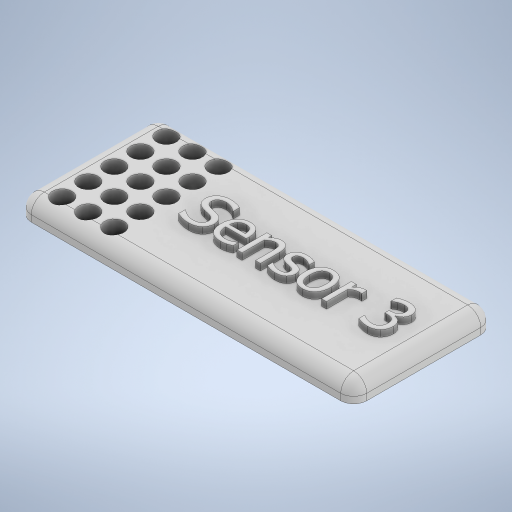
# Autodesk Inventor part: sensor3
Saved by Autodesk Inventor 2024 (Build 280153000, 153)
## iProperties
Created: 2024-03-06
Part Number: sensor3
Material: Generic
Document SubType Name: Modeling
Designer: quinten
Density: 1 g/cm^3
Appearance: Default
Author: quinten
Autodesk Inventor part; units mm, degrees
ref_plane "YZ Plane" through (0, 0, 0) normal (1, 0, 0) x (0, 1, 0)
ref_plane "XZ Plane" through (0, 0, 0) normal (0, 1, 0) x (-1, 0, 0)
ref_plane "XY Plane" through (0, 0, 0) normal (0, 0, 1) x (1, 0, 0)
sketch "Sketch1" plane through (0, 0, 0) normal (0, 1, 0) x (-1, 0, 0)
  line L0 (0, 0) -> (51.5, 0)
  line L1 (51.5, 0) -> (51.5, -21.5)
  line L2 (51.5, -21.5) -> (0, -21.5)
  line L3 (0, -21.5) -> (0, 0)
  line L4 (51.5, -10.75) -> (0, -10.75) construction
  line L5 (47.5, 0) -> (47.5, -21.5) construction
  circle A0 centre (47.5, -2.75) radius 1.5
  circle A1 centre (47.5, -10.75) radius 1.5
  circle A2 centre (47.5, -6.75) radius 1.5
  circle A3 centre (47.5, -14.75) radius 1.5
  circle A4 centre (47.5, -18.75) radius 1.5
  circle A5 centre (43.5, -2.75) radius 1.5
  circle A6 centre (43.5, -6.75) radius 1.5
  circle A7 centre (43.5, -10.75) radius 1.5
  circle A8 centre (43.5, -14.75) radius 1.5
  circle A9 centre (43.5, -18.75) radius 1.5
  circle A10 centre (39.5, -2.75) radius 1.5
  circle A11 centre (39.5, -6.75) radius 1.5
  circle A12 centre (39.5, -10.75) radius 1.5
  circle A13 centre (39.5, -14.75) radius 1.5
  circle A14 centre (39.5, -18.75) radius 1.5
  dimension "d0" = 51.5
  dimension "d1" = 21.5
  dimension "d2" = 4
  dimension "d3" = 3
  dimension "d4" = 3
  dimension "d5" = 3
  dimension "d6" = 3
  dimension "d7" = 3
  dimension "d8" = 4
  dimension "d9" = 4
  dimension "d10" = 4
  dimension "d11" = 4
  dimension "d14" = 4
  constraints: 15 centre point, 12 end point, 6 point on line, 3 midpoint, 2 horizontal, 2 parallel, 2 perpendicular, 20 other
  measures "d0" distance of L1.end L2.end
  measures "d1" distance of L0.end L1.end
  measures "d2" distance between parallel lines of L1 L5
  measures "d3" diameter of A0
  measures "d4" diameter of A1
  measures "d5" diameter of A2
  measures "d6" diameter of A3
  measures "d7" diameter of A4
  measures "d8" distance of A1.centre A3.centre
  measures "d9" distance of A3.centre A4.centre
  measures "d10" distance of A1.centre A2.centre
  measures "d11" distance of A2.centre A0.centre
  measures "d14" distance of A0.centre A5.centre
extrude "Extrusion1" add sketch "Sketch1" along normal blind 3
fillet "Fillet1" radius 2 8 edges at (0, 1.5, 0) (-25.75, 3, 0) (0, 3, -10.75) (0, 1.5, -21.5) (-25.75, 3, -21.5) (-51.5, 3, -10.75) (-51.5, 1.5, 0) (-51.5, 1.5, -21.5)
sketch "Sketch2" plane through (0, 3, 0) normal (0, 1, 0) x (1, 0, 0)
  line L0 (-35.6591, 14.3268) -> (-1.7873, 14.3268) construction
  line L1 (-1.7873, 14.3268) -> (-1.7873, 6.1649) construction
  line L2 (-1.7873, 6.1649) -> (-35.6591, 6.1649) construction
  line L3 (-35.6591, 6.1649) -> (-35.6591, 14.3268) construction
  spline S0 degree 2 poles (-33.3407, 7.9895) (-34.0031, 7.9895) (-34.9325, 8.2663) (-35.3428, 8.464) knots 0 0 0 1 2 2 2
  line L4 (-35.3428, 8.464) -> (-35.3428, 9.4823)
  line L5 (-35.3428, 9.4823) -> (-35.2834, 9.4823)
  spline S1 degree 2 poles (-35.2834, 9.4823) (-34.883, 9.1067) (-33.8697, 8.6914) (-33.4, 8.6914) knots 0 0 0 1 2 2 2
  spline S2 degree 2 poles (-33.4, 8.6914) (-32.7278, 8.6914) (-32.0406, 9.25) (-32.0406, 9.7097) knots 0 0 0 1 2 2 2
  spline S3 degree 2 poles (-32.0406, 9.7097) (-32.0406, 10.0755) (-32.4015, 10.5303) (-32.792, 10.644) knots 0 0 0 1 2 2 2
  spline S4 degree 2 poles (-32.792, 10.644) (-33.0738, 10.7231) (-33.5434, 10.8319) (-33.8944, 10.9208) knots 0 0 0 1 2 2 2
  spline S5 degree 2 poles (-33.8944, 10.9208) (-34.2107, 11.0049) (-34.71, 11.257) (-34.9028, 11.4597) knots 0 0 0 1 2 2 2
  spline S6 degree 2 poles (-34.9028, 11.4597) (-35.0906, 11.6623) (-35.2983, 12.2061) (-35.2983, 12.562) knots 0 0 0 1 2 2 2
  spline S7 degree 2 poles (-35.2983, 12.562) (-35.2983, 13.3035) (-34.1415, 14.307) (-33.2468, 14.307) knots 0 0 0 1 2 2 2
  spline S8 degree 2 poles (-33.2468, 14.307) (-32.7327, 14.307) (-31.8231, 14.1043) (-31.4326, 13.9115) knots 0 0 0 1 2 2 2
  line L6 (-31.4326, 13.9115) -> (-31.4326, 12.9426)
  line L7 (-31.4326, 12.9426) -> (-31.4919, 12.9426)
  spline S9 degree 2 poles (-31.4919, 12.9426) (-31.7836, 13.2096) (-32.6932, 13.605) (-33.1924, 13.605) knots 0 0 0 1 2 2 2
  spline S10 degree 2 poles (-33.1924, 13.605) (-33.756, 13.605) (-34.453, 13.0761) (-34.453, 12.646) knots 0 0 0 1 2 2 2
  spline S11 degree 2 poles (-34.453, 12.646) (-34.453, 12.2605) (-34.0427, 11.8007) (-33.6571, 11.6969) knots 0 0 0 1 2 2 2
  spline S12 degree 2 poles (-33.6571, 11.6969) (-33.4, 11.6277) (-32.6536, 11.4498) (-32.4064, 11.3756) knots 0 0 0 1 2 2 2
  spline S13 degree 2 poles (-32.4064, 11.3756) (-31.7787, 11.1828) (-31.1953, 10.4067) (-31.1953, 9.8383) knots 0 0 0 1 2 2 2
  spline S14 degree 2 poles (-31.1953, 9.8383) (-31.1953, 9.4774) (-31.487, 8.7853) (-31.749, 8.5431) knots 0 0 0 1 2 2 2
  spline S15 degree 2 poles (-31.749, 8.5431) (-32.0406, 8.2762) (-32.7821, 7.9895) (-33.3407, 7.9895) knots 0 0 0 1 2 2 2
  spline S16 degree 2 poles (-28.4419, 7.9944) (-29.5393, 7.9944) (-30.7455, 9.2253) (-30.7455, 10.3622) knots 0 0 0 1 2 2 2
  spline S17 degree 2 poles (-30.7455, 10.3622) (-30.7455, 11.4794) (-29.574, 12.8042) (-28.6298, 12.8042) knots 0 0 0 1 2 2 2
  spline S18 degree 2 poles (-28.6298, 12.8042) (-28.2047, 12.8042) (-27.5472, 12.5571) (-27.305, 12.2951) knots 0 0 0 1 2 2 2
  spline S19 degree 2 poles (-27.305, 12.2951) (-27.0578, 12.0331) (-26.7958, 11.2768) (-26.7958, 10.728) knots 0 0 0 1 2 2 2
  line L8 (-26.7958, 10.728) -> (-26.7958, 10.3079)
  line L9 (-26.7958, 10.3079) -> (-29.9645, 10.3079)
  spline S20 degree 2 poles (-29.9645, 10.3079) (-29.9645, 9.512) (-29.1637, 8.6667) (-28.4518, 8.6667) knots 0 0 0 1 2 2 2
  spline S21 degree 2 poles (-28.4518, 8.6667) (-28.1997, 8.6667) (-27.7103, 8.7804) (-27.5126, 8.8694) knots 0 0 0 1 2 2 2
  spline S22 degree 2 poles (-27.5126, 8.8694) (-27.305, 8.9682) (-27.0183, 9.1413) (-26.9244, 9.2204) knots 0 0 0 1 2 2 2
  line L10 (-26.9244, 9.2204) -> (-26.8799, 9.2204)
  line L11 (-26.8799, 9.2204) -> (-26.8799, 8.38)
  spline S23 degree 2 poles (-26.8799, 8.38) (-27.0133, 8.3256) (-27.4187, 8.1674) (-27.5769, 8.1229) knots 0 0 0 1 2 2 2
  spline S24 degree 2 poles (-27.5769, 8.1229) (-27.7993, 8.0587) (-28.1651, 7.9944) (-28.4419, 7.9944) knots 0 0 0 1 2 2 2
  spline S25 degree 2 poles (-27.5472, 10.8961) (-27.5571, 11.2075) (-27.6856, 11.6623) (-27.8092, 11.8156) knots 0 0 0 1 2 2 2
  spline S26 degree 2 poles (-27.8092, 11.8156) (-27.9427, 11.9886) (-28.3628, 12.1715) (-28.6743, 12.1715) knots 0 0 0 1 2 2 2
  spline S27 degree 2 poles (-28.6743, 12.1715) (-28.9808, 12.1715) (-29.4108, 11.9886) (-29.5888, 11.8106) knots 0 0 0 1 2 2 2
  spline S28 degree 2 poles (-29.5888, 11.8106) (-29.7618, 11.6277) (-29.9398, 11.1878) (-29.9645, 10.8961) knots 0 0 0 1 2 2 2
  line L12 (-29.9645, 10.8961) -> (-27.5472, 10.8961)
  line L13 (-22.421, 8.0982) -> (-23.1922, 8.0982)
  line L14 (-23.1922, 8.0982) -> (-23.1922, 10.7083)
  spline S29 degree 2 poles (-23.1922, 10.7083) (-23.1922, 11.0246) (-23.2515, 11.5684) (-23.3405, 11.7315) knots 0 0 0 1 2 2 2
  spline S30 degree 2 poles (-23.3405, 11.7315) (-23.4344, 11.9045) (-23.7705, 12.0726) (-24.0573, 12.0726) knots 0 0 0 1 2 2 2
  spline S31 degree 2 poles (-24.0573, 12.0726) (-24.344, 12.0726) (-24.952, 11.7661) (-25.2436, 11.519) knots 0 0 0 1 2 2 2
  line L15 (-25.2436, 11.519) -> (-25.2436, 8.0982)
  line L16 (-25.2436, 8.0982) -> (-26.0148, 8.0982)
  line L17 (-26.0148, 8.0982) -> (-26.0148, 12.6757)
  line L18 (-26.0148, 12.6757) -> (-25.2436, 12.6757)
  line L19 (-25.2436, 12.6757) -> (-25.2436, 12.1665)
  spline S32 degree 2 poles (-25.2436, 12.1665) (-24.8976, 12.478) (-24.2303, 12.8042) (-23.8546, 12.8042) knots 0 0 0 1 2 2 2
  spline S33 degree 2 poles (-23.8546, 12.8042) (-23.1823, 12.8042) (-22.421, 11.9144) (-22.421, 11.0691) knots 0 0 0 1 2 2 2
  line L20 (-22.421, 11.0691) -> (-22.421, 8.0982)
  spline S34 degree 2 poles (-20.1026, 7.9895) (-20.5624, 7.9895) (-21.3582, 8.2366) (-21.6202, 8.3751) knots 0 0 0 1 2 2 2
  line L21 (-21.6202, 8.3751) -> (-21.6202, 9.2401)
  line L22 (-21.6202, 9.2401) -> (-21.5807, 9.2401)
  spline S35 degree 2 poles (-21.5807, 9.2401) (-21.4818, 9.161) (-21.2149, 8.9732) (-20.9924, 8.8694) knots 0 0 0 1 2 2 2
  spline S36 degree 2 poles (-20.9924, 8.8694) (-20.7996, 8.7755) (-20.3251, 8.637) (-20.073, 8.637) knots 0 0 0 1 2 2 2
  spline S37 degree 2 poles (-20.073, 8.637) (-19.8901, 8.637) (-19.4699, 8.7211) (-19.371, 8.7903) knots 0 0 0 1 2 2 2
  spline S38 degree 2 poles (-19.371, 8.7903) (-19.2277, 8.8842) (-19.0992, 9.0968) (-19.0992, 9.3143) knots 0 0 0 1 2 2 2
  spline S39 degree 2 poles (-19.0992, 9.3143) (-19.0992, 9.5862) (-19.3957, 9.8679) (-19.7764, 9.9618) knots 0 0 0 1 2 2 2
  spline S40 degree 2 poles (-19.7764, 9.9618) (-19.9247, 9.9964) (-20.3992, 10.0953) (-20.6019, 10.1497) knots 0 0 0 1 2 2 2
  spline S41 degree 2 poles (-20.6019, 10.1497) (-21.1259, 10.3029) (-21.6005, 10.9357) (-21.6005, 11.3855) knots 0 0 0 1 2 2 2
  spline S42 degree 2 poles (-21.6005, 11.3855) (-21.6005, 12.0084) (-20.6662, 12.7845) (-19.895, 12.7845) knots 0 0 0 1 2 2 2
  spline S43 degree 2 poles (-19.895, 12.7845) (-19.5144, 12.7845) (-18.7432, 12.5966) (-18.4812, 12.4533) knots 0 0 0 1 2 2 2
  line L23 (-18.4812, 12.4533) -> (-18.4812, 11.6277)
  line L24 (-18.4812, 11.6277) -> (-18.5208, 11.6277)
  spline S44 degree 2 poles (-18.5208, 11.6277) (-18.8174, 11.865) (-19.5391, 12.1369) (-19.9099, 12.1369) knots 0 0 0 1 2 2 2
  spline S45 degree 2 poles (-19.9099, 12.1369) (-20.2905, 12.1369) (-20.8145, 11.8156) (-20.8145, 11.4943) knots 0 0 0 1 2 2 2
  spline S46 degree 2 poles (-20.8145, 11.4943) (-20.8145, 11.2026) (-20.503, 10.9208) (-20.157, 10.8319) knots 0 0 0 1 2 2 2
  spline S47 degree 2 poles (-20.157, 10.8319) (-19.9889, 10.7874) (-19.5638, 10.6984) (-19.3315, 10.644) knots 0 0 0 1 2 2 2
  spline S48 degree 2 poles (-19.3315, 10.644) (-18.8273, 10.5155) (-18.3132, 9.9272) (-18.3132, 9.4181) knots 0 0 0 1 2 2 2
  spline S49 degree 2 poles (-18.3132, 9.4181) (-18.3132, 9.1215) (-18.5455, 8.5975) (-18.7729, 8.4047) knots 0 0 0 1 2 2 2
  spline S50 degree 2 poles (-18.7729, 8.4047) (-19.0151, 8.202) (-19.633, 7.9895) (-20.1026, 7.9895) knots 0 0 0 1 2 2 2
  spline S51 degree 2 poles (-13.8346, 10.387) (-13.8346, 9.2302) (-14.9468, 7.9697) (-15.8761, 7.9697) knots 0 0 0 1 2 2 2
  spline S52 degree 2 poles (-15.8761, 7.9697) (-16.8302, 7.9697) (-17.9227, 9.2698) (-17.9227, 10.387) knots 0 0 0 1 2 2 2
  spline S53 degree 2 poles (-17.9227, 10.387) (-17.9227, 11.5338) (-16.7956, 12.8042) (-15.8761, 12.8042) knots 0 0 0 1 2 2 2
  spline S54 degree 2 poles (-15.8761, 12.8042) (-14.9468, 12.8042) (-13.8346, 11.5387) (-13.8346, 10.387) knots 0 0 0 1 2 2 2
  spline S55 degree 2 poles (-14.6304, 10.387) (-14.6304, 11.2768) (-15.278, 12.1418) (-15.8761, 12.1418) knots 0 0 0 1 2 2 2
  spline S56 degree 2 poles (-15.8761, 12.1418) (-16.4743, 12.1418) (-17.1268, 11.2768) (-17.1268, 10.387) knots 0 0 0 1 2 2 2
  spline S57 degree 2 poles (-17.1268, 10.387) (-17.1268, 9.5219) (-16.4743, 8.6321) (-15.8761, 8.6321) knots 0 0 0 1 2 2 2
  spline S58 degree 2 poles (-15.8761, 8.6321) (-15.2829, 8.6321) (-14.6304, 9.5071) (-14.6304, 10.387) knots 0 0 0 1 2 2 2
  line L25 (-10.6165, 11.8502) -> (-10.656, 11.8502)
  spline S59 degree 2 poles (-10.656, 11.8502) (-10.745, 11.8749) (-10.9378, 11.8848) (-11.0713, 11.8848) knots 0 0 0 1 2 2 2
  spline S60 degree 2 poles (-11.0713, 11.8848) (-11.3827, 11.8848) (-11.9957, 11.6129) (-12.2725, 11.346) knots 0 0 0 1 2 2 2
  line L26 (-12.2725, 11.346) -> (-12.2725, 8.0982)
  line L27 (-12.2725, 8.0982) -> (-13.0436, 8.0982)
  line L28 (-13.0436, 8.0982) -> (-13.0436, 12.6757)
  line L29 (-13.0436, 12.6757) -> (-12.2725, 12.6757)
  line L30 (-12.2725, 12.6757) -> (-12.2725, 11.9935)
  spline S61 degree 2 poles (-12.2725, 11.9935) (-11.8523, 12.3692) (-11.2245, 12.6757) (-10.9279, 12.6757) knots 0 0 0 1 2 2 2
  spline S62 degree 2 poles (-10.9279, 12.6757) (-10.8093, 12.6757) (-10.6906, 12.6658) (-10.6165, 12.651) knots 0 0 0 1 2 2 2
  line L31 (-10.6165, 12.651) -> (-10.6165, 11.8502)
  spline S63 degree 2 poles (-5.866, 13.6199) (-6.0885, 13.6199) (-6.5284, 13.5111) (-6.741, 13.4271) knots 0 0 0 1 2 2 2
  spline S64 degree 2 poles (-6.741, 13.4271) (-6.9387, 13.343) (-7.2304, 13.1651) (-7.344, 13.086) knots 0 0 0 1 2 2 2
  line L32 (-7.344, 13.086) -> (-7.3935, 13.086)
  line L33 (-7.3935, 13.086) -> (-7.3935, 13.9511)
  spline S65 degree 2 poles (-7.3935, 13.9511) (-7.1265, 14.0944) (-6.212, 14.3268) (-5.8017, 14.3268) knots 0 0 0 1 2 2 2
  spline S66 degree 2 poles (-5.8017, 14.3268) (-5.3865, 14.3268) (-4.7686, 14.1587) (-4.5165, 13.9807) knots 0 0 0 1 2 2 2
  spline S67 degree 2 poles (-4.5165, 13.9807) (-4.2496, 13.7879) (-3.9727, 13.2293) (-3.9727, 12.8537) knots 0 0 0 1 2 2 2
  spline S68 degree 2 poles (-3.9727, 12.8537) (-3.9727, 12.3494) (-4.6351, 11.5882) (-5.0998, 11.4893) knots 0 0 0 1 2 2 2
  line L34 (-5.0998, 11.4893) -> (-5.0998, 11.43)
  spline S69 degree 2 poles (-5.0998, 11.43) (-4.907, 11.3904) (-4.4671, 11.2125) (-4.2792, 11.0345) knots 0 0 0 1 2 2 2
  spline S70 degree 2 poles (-4.2792, 11.0345) (-4.0914, 10.8615) (-3.8541, 10.3079) (-3.8541, 9.9075) knots 0 0 0 1 2 2 2
  spline S71 degree 2 poles (-3.8541, 9.9075) (-3.8541, 9.4972) (-4.1359, 8.8002) (-4.3929, 8.5332) knots 0 0 0 1 2 2 2
  spline S72 degree 2 poles (-4.3929, 8.5332) (-4.6599, 8.2564) (-5.4162, 7.9697) (-5.8957, 7.9697) knots 0 0 0 1 2 2 2
  spline S73 degree 2 poles (-5.8957, 7.9697) (-6.3554, 7.9697) (-7.2551, 8.1921) (-7.5616, 8.3454) knots 0 0 0 1 2 2 2
  line L35 (-7.5616, 8.3454) -> (-7.5616, 9.2105)
  line L36 (-7.5616, 9.2105) -> (-7.5022, 9.2105)
  spline S74 degree 2 poles (-7.5022, 9.2105) (-7.2452, 9.0226) (-6.3752, 8.6766) (-5.9451, 8.6766) knots 0 0 0 1 2 2 2
  spline S75 degree 2 poles (-5.9451, 8.6766) (-5.693, 8.6766) (-5.1888, 8.8348) (-5.0207, 9.0177) knots 0 0 0 1 2 2 2
  spline S76 degree 2 poles (-5.0207, 9.0177) (-4.8576, 9.2006) (-4.6846, 9.6356) (-4.6846, 9.9668) knots 0 0 0 1 2 2 2
  spline S77 degree 2 poles (-4.6846, 9.9668) (-4.6846, 10.298) (-4.8774, 10.728) (-5.0504, 10.8516) knots 0 0 0 1 2 2 2
  spline S78 degree 2 poles (-5.0504, 10.8516) (-5.2234, 10.9752) (-5.693, 11.0691) (-5.9698, 11.0691) knots 0 0 0 1 2 2 2
  line L37 (-5.9698, 11.0691) -> (-6.3158, 11.0691)
  line L38 (-6.3158, 11.0691) -> (-6.3158, 11.7464)
  line L39 (-6.3158, 11.7464) -> (-6.044, 11.7464)
  spline S79 degree 2 poles (-6.044, 11.7464) (-5.4953, 11.7464) (-4.8032, 12.2704) (-4.8032, 12.7696) knots 0 0 0 1 2 2 2
  spline S80 degree 2 poles (-4.8032, 12.7696) (-4.8032, 13.002) (-4.9812, 13.3332) (-5.1245, 13.432) knots 0 0 0 1 2 2 2
  spline S81 degree 2 poles (-5.1245, 13.432) (-5.2778, 13.5358) (-5.6534, 13.6199) (-5.866, 13.6199) knots 0 0 0 1 2 2 2
  point P0 (0, 0)
  constraints: 2 other
extrude "Extrusion2" add sketch "Sketch2" along normal blind 1
equation "\"d2\" = d9"
equation "\"d3\" = d7"
equation "\"d4\" = d7"
equation "\"d5\" = d7"
equation "\"d6\" = d7"
equation "\"d9\" = d8"
equation "\"d10\" = d9"
equation "\"d11\" = d10"
body "Solid1"
